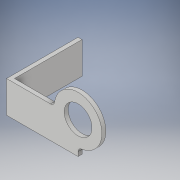
# Autodesk Inventor part: Pivot Bracket
Saved by Autodesk Inventor 2017 (Build 210142000, 142)
## iProperties
Created: 2017-06-10
Part Number: Pivot Bracket
Material: Generic
Document SubType Name: Modeling
Designer: Matthew
Density: 1 g/cm^3
Appearance: Default
Author: Matthew
Autodesk Inventor part; units mm, degrees
ref_plane "YZ Plane" through (0, 0, 0) normal (1, 0, 0) x (0, 1, 0)
ref_plane "XZ Plane" through (0, 0, 0) normal (0, 1, 0) x (-1, 0, 0)
ref_plane "XY Plane" through (0, 0, 0) normal (0, 0, 1) x (1, 0, 0)
sketch "Sketch1" plane through (0, 0, 0) normal (0, 1, 0) x (-1, 0, 0)
  line L0 (0, 0) -> (57.15, 0)
  line L1 (112.534, 31.2241) -> (58.0687, -3.175)
  line L2 (58.0687, -3.175) -> (0, -3.175)
  line L3 (0, -3.175) -> (0, 0)
  line L4 (110.8385, 33.9086) -> (112.534, 31.2241)
  line L5 (57.15, 0) -> (110.8385, 33.9086)
  dimension "d0" = 3.175
  dimension "d1" = 3.175
  dimension "d3" = 57.15
  dimension "d4" = 63.5
  dimension "d5" = 147.724
  constraints: 12 end point, 2 parallel, 2 perpendicular, 1 horizontal
  measures "d0" distance of L2.end L0.start
  measures "d1" distance of L4.start L1.start
  measures "d3" distance of L0.start L0.end
  measures "d4" distance of L0.end L4.start
  measures "d5" angle of L0 L5
extrude "Extrusion1" add sketch "Sketch1" along normal blind 25.4
sketch "Sketch2" plane through (-57.15, 0, 0) normal (0, 0, 1) x (1, 0, 0)
  line L0 (0, 25.4) -> (57.15, 25.4) projected
  circle A0 centre (57.15, 25.4) radius 11.1125
  line L1 (57.15, 0) -> (57.15, 25.4) projected
  circle A1 centre (57.15, 25.4) radius 19.05
  dimension "d8" = 22.225
  dimension "d9" = 38.1
  constraints: 2 centre point, 1 coincident
  measures "d8" diameter of A0
  measures "d9" diameter of A1
extrude "Extrusion2" add sketch "Sketch2" against normal blind 3.175 contours A1 L1 A0 L0 | L0 A0 L1 A1
sketch "Sketch3" plane through (-57.15, 0, 0) normal (0, 0, 1) x (1, 0, 0)
  line L0 (57.15, 14.2875) -> (57.15, 25.4) projected
  circle A0 centre (57.15, 25.4) radius 11.1125
  point P0 (57.15, 0)
  constraints: 1 vertical alignment, 2 other
extrude "Extrusion3" cut sketch "Sketch3" against normal blind 3.175
fillet "Fillet1" radius 3.175 2 edges at (0, 6.35, -1.5875) (-19.05, 25.4, -1.5875)
sketch "Sketch4" plane through (0, 25.4, 0) normal (0, 1, 0) x (1, 0, 0)
  line L0 (0, 0) -> (-63.5, 0)
  line L1 (-136.491, 61.8746) -> (-57.15, 61.8746)
  line L2 (-57.15, 61.8746) -> (-57.15, -40.3817)
  line L3 (-57.15, -40.3817) -> (-136.491, -40.3817)
  line L4 (-136.491, -40.3817) -> (-136.491, 61.8746)
  dimension "d15" = 63.5
  constraints: 10 end point, 2 horizontal, 2 parallel, 1 perpendicular
  measures "d15" distance of L0.start L0.end
extrude "Extrusion4" cut sketch "Sketch4" against normal blind 31.75
sketch "Sketch5" plane through (0, 25.4, 0) normal (0, 1, 0) x (1, 0, 0)
  line L0 (0, 0) -> (-57.15, 0)
  line L1 (-57.15, 0) -> (-57.15, 3.175) projected
  line L2 (-57.15, 0) -> (-53.975, 0)
  line L3 (-53.975, 0) -> (-53.975, 57.15)
  line L4 (-53.975, 57.15) -> (-57.15, 57.15)
  line L5 (-57.15, 57.15) -> (-57.15, 0)
  dimension "d18" = 57.15
  dimension "d19" = 3.175
  dimension "d20" = 57.15
  constraints: 10 end point, 2 horizontal, 2 parallel, 1 perpendicular
  measures "d18" distance of L0.start L0.end
  measures "d19" distance of L4.end L3.end
  measures "d20" distance of L3.end L2.end
extrude "Extrusion5" add sketch "Sketch5" against normal up to surface (25.4 mm away)
body "Solid1"
